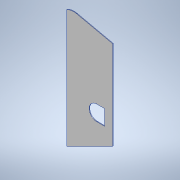
# Autodesk Inventor part: pokrywa prawa
Saved by Autodesk Inventor 2022.3 (Build 263350000, 350)
## iProperties
Created: 2022-10-11
Part Number: pokrywa prawa
Material: Aluminum 6061
Document SubType Name: Modeling
Designer: komputer
Density: 2.7 g/cm^3
Appearance: Aluminum - Flat
Author: komputer
Autodesk Inventor part; units mm, degrees
ref_plane "YZ Plane" through (0, 0, 0) normal (1, 0, 0) x (0, 1, 0)
ref_plane "XZ Plane" through (0, 0, 0) normal (0, 1, 0) x (-1, 0, 0)
ref_plane "XY Plane" through (0, 0, 0) normal (0, 0, 1) x (1, 0, 0)
sketch "Sketch1" plane through (0, 0, 0) normal (0, 0, 1) x (1, 0, 0)
  line L0 (-17.5, -33.2499) -> (-17.5, 57.9837) projected
  arc A0 (-10.0449, 58.8745) -> (-17.5, 57.9837) centre (-12.5, 47.7794) ccw projected
  line L1 (-10.0449, 58.8745) -> (17.5, 52.7794) projected
  line L2 (17.5, 52.7794) -> (17.5, -15.7501) projected
  line L3 (17.5, -15.7501) -> (-17.5, -33.2499) projected
  line L4 (0.5, 7.1892) -> (0.5, 22.231) projected
  line L5 (0.5, 22.231) -> (-5.8925, 22.231) projected
  line L6 (-5.8925, 22.231) -> (-5.8925, 7.1892) projected
  line L7 (-5.8925, 7.1892) -> (0.5, 7.1892) projected
  point P0 (0, 0)
extrude "Extrusion1" add sketch "Sketch1" along normal blind 0.5 contours L0 A0 L1 L2 L3 | L7 L6 L5 L4
sketch "Sketch2" plane through (0, 0, 0.5) normal (0, 0, 1) x (1, 0, 0)
  circle A0 centre (-7.1425, -8.6154) radius 1.25 projected
  circle A1 centre (-5.3255, 26.728) radius 1.25 projected
  circle A2 centre (12, 26.728) radius 1.25 projected
  line L0 (4.8837, -12.3662) -> (-3.9853, -13.2144) projected
  line L1 (-3.9853, -13.2144) -> (-3.2796, -20.5939) projected
  line L2 (-3.2796, -20.5939) -> (-5.5333, -16.0863) projected
  line L3 (-5.5333, -16.0863) -> (-14.5107, -20.575) projected
  line L4 (-14.5107, -20.575) -> (-10.0386, -29.5193) projected
  line L5 (-10.0386, -29.5193) -> (-14.6056, -31.8027) projected
  arc A3 (-17.5, -30.0139) -> (-14.6056, -31.8027) centre (-15.5, -30.0139) ccw projected
  line L6 (-17.5, -30.0139) -> (-17.5, -1.8864) projected
  line L7 (-17.5, -1.8864) -> (-7.5, -1.8864) projected
  line L8 (-7.5, -1.8864) -> (-7.5, 7.5751) projected
  line L9 (-7.5, 7.5751) -> (-8.8, 7.5751) projected
  line L10 (-8.8, 26.3195) -> (-8.8, 7.5751) projected
  spline S0 degree 3 poles (-14.2046, 28.2052) (-13.4118, 28.2052) (-12.6544, 28.0226) (-10.9379, 27.4679) (-9.8551, 26.8958) (-8.8077, 26.3237) (-8.8038, 26.3216) (-8.8, 26.3195) knots -0.001308 -0.001308 -0.001308 -0.001308 0.187612 0.187612 0.544344 0.544344 0.545652 0.545652 0.545652 0.545652 projected
  line L11 (-14.2046, 28.2052) -> (-17.5, 28.2052) projected
  line L12 (-17.5, 28.2052) -> (-17.5, 31.9794) projected
  arc A4 (-17.5, 31.9794) -> (-4.376, 33.2499) centre (-12.5, 48.7499) ccw projected
  arc A5 (-4.376, 33.2499) -> (2.7674, 54.4137) centre (-12.5, 47.7794) ccw projected
  arc A6 (3.9006, 55.7887) -> (2.7674, 54.4137) centre (3.6845, 54.8123) ccw projected
  line L13 (3.9006, 55.7887) -> (16.7161, 52.9529) projected
  arc A7 (17.5, 51.9765) -> (16.7161, 52.9529) centre (16.5, 51.9765) ccw projected
  line L14 (17.5, 51.9765) -> (17.5, 7.0459) projected
  line L15 (17.5, 7.0459) -> (5.1606, 7.0459) projected
  line L16 (5.1606, 7.0459) -> (5.1606, 20.2725) projected
  arc A8 (5.1606, 20.2725) -> (-1.3191, 20.2725) centre (1.9208, 20.2725) ccw projected
  line L17 (-1.3191, 20.2725) -> (-1.3191, 3.7386) projected
  arc A9 (-1.321, 3.6769) -> (-1.3191, 3.7386) centre (-2.3191, 3.7386) ccw projected
  line L18 (-1.321, 3.6769) -> (-1.623, -1.2058) projected
  arc A10 (-1.623, -1.2058) -> (-1.1883, -2.0937) centre (-0.6249, -1.2675) ccw projected
  line L19 (-1.1883, -2.0937) -> (4.4471, -5.9368) projected
  arc A11 (4.8837, -6.7629) -> (4.4471, -5.9368) centre (3.8837, -6.7629) ccw projected
  line L20 (4.8837, -6.7629) -> (4.8837, -12.3662) projected
  line L21 (-17.5, 57.9837) -> (-17.5, -33.2499) projected
  line L22 (-17.5, -33.2499) -> (17.5, -15.7501) projected
  line L23 (17.5, -15.7501) -> (17.5, 52.7794) projected
  line L24 (17.5, 52.7794) -> (-10.0449, 58.8745) projected
  arc A12 (-10.0449, 58.8745) -> (-17.5, 57.9837) centre (-12.5, 47.7794) ccw projected
  line L25 (5.1606, 7.0459) -> (-1.321, 3.6769)
  line L26 (4.7678, -6.2957) -> (11.3303, -6.2957)
  line L27 (11.3303, -6.2957) -> (11.3303, 7.0459)
  circle A13 centre (5.4296, 0.5354) radius 5.9007
  line L28 (5.4296, 0.5354) -> (11.3303, 0.5354)
  line L29 (11.3303, 0.5354) -> (11.3303, 6.4362)
  line L30 (11.3303, 6.4362) -> (5.4296, 6.4362)
  line L31 (5.4296, 6.4362) -> (5.4296, 0.5354)
  line L32 (11.3303, 0.5354) -> (5.4296, 0.5354)
  line L33 (5.4296, 0.5354) -> (5.4296, -5.3653)
  line L34 (5.4296, -5.3653) -> (11.3303, -5.3653)
  line L35 (11.3303, -5.3653) -> (11.3303, 0.5354)
  point P0 (0, 0)
  constraints: 22 end point, 4 parallel, 3 horizontal, 3 point on line, 2 perpendicular, 1 midpoint, 1 point on circle, 1 vertical, 5 other
extrude "Extrusion2" cut sketch "Sketch2" against normal blind 10 contours A13 L31 L33 | L34 A13 L27 | L33 L28 A13 | A13 L30 L27 | L28 L31 A13
body "Solid1"
